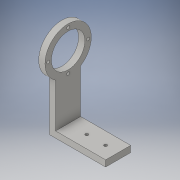
# Autodesk Inventor part: LED Hinge
Saved by Autodesk Inventor 2016 (Build 200138000, 138)
## iProperties
Created: 2017-09-28
Part Number: LED Hinge
Material: Generic
Document SubType Name: Modeling
Designer: Student
Density: 1 g/cm^3
Appearance: Default
Author: Student
Autodesk Inventor part; units mm, degrees
ref_plane "YZ Plane" through (0, 0, 0) normal (1, 0, 0) x (0, 1, 0)
ref_plane "XZ Plane" through (0, 0, 0) normal (0, 1, 0) x (-1, 0, 0)
ref_plane "XY Plane" through (0, 0, 0) normal (0, 0, 1) x (1, 0, 0)
sketch "Sketch1" plane through (0, 0, 0) normal (1, 0, 0) x (0, 1, 0)
  circle A0 centre (0, 0) radius 17.018
  circle A1 centre (0, 0) radius 23.495
  line L0 (-19.7668, 12.7) -> (-70.7247, 12.7)
  line L1 (-70.7247, 12.7) -> (-70.7247, -12.7)
  line L2 (-70.7247, -12.7) -> (-19.7668, -12.7)
  dimension "d0" = 6.477
  dimension "d1" = 34.036
  dimension "d7" = 25.4
  constraints: 6 end point, 2 centre point, 2 coincident, 2 horizontal, 2 point on circle, 1 perpendicular
  measures "d0" radial gap between concentric circles of A1 A0
  measures "d1" diameter of A0
  measures "d7" distance of L0.end L1.end
extrude "Extrusion1" add sketch "Sketch1" along normal blind 6.35
sketch "Sketch2" plane through (6.35, 0, 0) normal (1, 0, 0) x (0, 0, -1)
  line L0 (-12.7, -19.7668) -> (-12.7, -70.7247) projected
  line L1 (12.7, -70.7247) -> (12.7, -19.7668) projected
  line L2 (-12.7, -70.7247) -> (12.7, -70.7247)
  line L3 (12.7, -70.7247) -> (12.7, -64.3747)
  line L4 (12.7, -64.3747) -> (-12.7, -64.3747)
  line L5 (-12.7, -64.3747) -> (-12.7, -70.7247)
  point P0 (0, 0)
  dimension "d10" = 6.35
  constraints: 8 end point, 2 parallel, 1 horizontal, 1 perpendicular, 1 point on line
  measures "d10" distance between parallel lines of L2 L4
extrude "Extrusion2" add sketch "Sketch2" along normal blind 50.8
sketch "Sketch3" plane through (0, -70.7247, -12.7) normal (0, -1, 0) x (1, 0, 0)
  circle A0 centre (25.4, 12.7) radius 1.5
  circle A1 centre (44.45, 12.7) radius 1.5
  line L0 (0, 25.4) -> (57.15, 25.4) projected
  line L1 (57.15, 25.4) -> (57.15, 0) projected
  line L2 (0, 25.4) -> (0, 0) projected
  point P0 (0, 12.7)
  dimension "d14" = 12.7
  dimension "d15" = 12.7
  dimension "d16" = 3
  dimension "d17" = 3
  dimension "d18" = 12.7
  dimension "d19" = 25.4
  constraints: 2 centre point
  measures "d14" distance from line of A0.centre L0
  measures "d15" distance from line of A1.centre L0
  measures "d16" diameter of A1
  measures "d17" diameter of A0
  measures "d18" distance from line of A1.centre L1
  measures "d19" distance from line of A0.centre L2
extrude "Extrusion3" cut sketch "Sketch3" against normal blind 50.8
sketch "Sketch4" plane through (6.35, 0, 0) normal (1, 0, 0) x (0, 0, -1)
  line L0 (0, 23.4884) -> (0, 17.018)
  circle A0 centre (0, 0) radius 17.018 projected
  circle A1 centre (0, 20.2532) radius 1.5
  circle A2 centre (-20.2532, 0) radius 1.5
  circle A3 centre (0, -20.2532) radius 1.5
  circle A4 centre (20.2532, 0) radius 1.5
  dimension "d22" = 3
  dimension "d25" = 360
  constraints: 4 centre point, 2 end point, 1 midpoint, 1 vertical, 1 vertical alignment, 10 other
  measures "d22" diameter of A1
extrude "Extrusion4" cut sketch "Sketch4" against normal blind 50.8 contours A1 L0 | L0 A1 | A2 | A3 | A4
body "Solid1"
